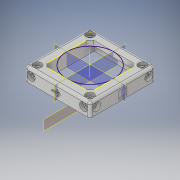
# Autodesk Inventor part: 10_Lid_v0_B
Saved by Autodesk Inventor 2019 (Build 230136000, 136)
## iProperties
Created: 2018-05-19
Part Number: 10_Lid_v0_B
Material: Generisch
Document SubType Name: Modeling
Designer: diederichbenedict
Density: 1 g/cm^3
Appearance: Vorgabe
Author: diederichbenedict
Autodesk Inventor part; units mm, degrees
ref_plane "YZ Plane" through (0, 0, 0) normal (1, 0, 0) x (0, 1, 0)
ref_plane "XZ Plane" through (0, 0, 0) normal (0, 1, 0) x (-1, 0, 0)
sketch "Skizze1" plane through (0, 0, 0) normal (0, 0, 1) x (1, 0, 0)
  line L0 (-3.2746, 3.2746) -> (46.5254, 3.2746)
  line L1 (46.5254, 3.2746) -> (46.5254, -46.5254)
  line L2 (46.5254, -46.5254) -> (-3.2746, -46.5254)
  line L3 (-3.2746, -46.5254) -> (-3.2746, 3.2746)
  line L4 (-3.2746, 3.2746) -> (46.5254, -46.5254) construction
  line L5 (46.5254, 3.2746) -> (-3.2746, -46.5254) construction
  line L6 (6.7254, -3.7254) -> (36.5254, -3.7254)
  line L7 (39.5254, -6.7254) -> (39.5254, -36.5254)
  line L8 (36.5254, -39.5254) -> (6.7254, -39.5254)
  line L9 (3.7254, -36.5254) -> (3.7254, -6.7254)
  line L10 (3.7254, -3.7254) -> (39.5254, -39.5254) construction
  line L11 (39.5254, -3.7254) -> (3.7254, -39.5254) construction
  line L12 (36.5254, -39.5254) -> (39.5254, -36.5254)
  line L13 (6.7254, -39.5254) -> (3.7254, -36.5254)
  line L14 (3.7254, -6.7254) -> (6.7254, -3.7254)
  line L15 (36.5254, -3.7254) -> (39.5254, -6.7254)
  line L16 (6.9985, -0.5594) -> (36.2523, -0.5594) projected
  line L17 (36.2523, -0.5594) -> (36.2523, 3.2746) projected
  line L18 (36.2523, 3.2746) -> (6.9985, 3.2746) projected
  line L19 (6.9985, 3.2746) -> (6.9985, -0.5594) projected
  point P0 (21.6254, -21.6254)
  point P1 (21.6254, -21.6254)
  dimension "d17" = 35.8
  dimension "d18" = 35.8
  dimension "d19" = 3
  dimension "d20" = 3
  dimension "d21" = 3
  dimension "d22" = 3
  dimension "d23" = 3
  dimension "d24" = 3
  dimension "d25" = 3
  dimension "d26" = 3
  constraints: 32 end point, 8 point on line, 5 midpoint, 4 parallel, 2 horizontal, 2 perpendicular
  measures "d17" distance of L10.end L11.end
  measures "d18" distance of L11.start L10.end
  measures "d19" distance of L8.start L10.end
  measures "d20" distance of L7.end L10.end
  measures "d21" distance of L8.end L11.end
  measures "d22" distance of L9.start L11.end
  measures "d23" distance of L9.end L10.start
  measures "d24" distance of L6.start L10.start
  measures "d25" distance of L6.end L11.start
  measures "d26" distance of L7.start L11.start
extrude "Extrusion1" add sketch "Skizze1" along normal blind 10.3
sketch "Skizze2" plane through (0, 0, 10.3) normal (0, 0, 1) x (1, 0, 0)
  arc A0 (41.4389, -3.1137) -> (40.137, -1.8118) centre (41.6254, -1.6254) ccw projected
  arc A1 (40.137, -41.4389) -> (41.4389, -40.137) centre (41.6254, -41.6254) ccw projected
  arc A2 (1.8118, -40.137) -> (3.1137, -41.4389) centre (1.6254, -41.6254) ccw projected
  arc A3 (3.1137, -1.8118) -> (1.8118, -3.1137) centre (1.6254, -1.6254) ccw projected
hole "Bohrung1" at (41.6254, -41.6254, 10.3) at (1.6254, -41.6254, 10.3) at (1.6254, -1.6254, 10.3) at (41.6254, -1.6254, 10.3) direction (0, 0, -1) diameter 3 end through all counterbore diameter 6 counterbore depth 2.5
fillet "Rundung1" radius 2 8 edges at (21.6254, -46.5254, 10.3) (-3.2746, -21.6254, 10.3) (21.6254, 3.2746, 10.3) (46.5254, -21.6254, 10.3) (46.5254, 3.2746, 5.15) (46.5254, -46.5254, 5.15) (-3.2746, -46.5254, 5.15) (-3.2746, 3.2746, 5.15)
sketch "Skizze3" plane through (-1.2746, -46.5254, 0) normal (0, -1, 0) x (1, 0, 0)
  line L0 (45.8, -37.7) -> (43.681, -37.7) construction
  line L1 (45.8, -35.7954) -> (45.8, -37.7) construction
  arc A0 (43.681, -37.7) -> (45.8, -35.7954) centre (42.9, -34.7) ccw projected
  line L2 (42.9, -36) -> (2.9, -36) construction
  line L3 (2.9, -36) -> (2.9, 5.3) construction
  line L4 (2.9, 5.3) -> (42.9, 5.3) construction
  line L5 (42.9, 5.3) -> (42.9, -36) construction
  dimension "d40" = 40
  dimension "d42" = 40
  constraints: 8 end point, 2 parallel, 1 horizontal, 1 perpendicular
  measures "d40" distance of L3.end L4.end
  measures "d42" distance from line of L4 A0.centre
sketch "Skizze4" plane through (0, 0, 10.3) normal (0, 0, 1) x (1, 0, 0)
  line L0 (36.5254, -39.5254) -> (6.7254, -39.5254) projected
  line L1 (39.5254, -6.7254) -> (39.5254, -36.5254) projected
  line L2 (3.7254, -36.5254) -> (3.7254, -6.7254) projected
  circle A0 centre (21.6254, -21.6254) radius 17.9
  point P0 (0, 0)
  constraints: 3 tangent, 1 centre point
ref_plane "Arbeitsebene1" through (3.7254, -5.5842, -33.1) normal (1, 0, 0) x (0, 1, 0)
sketch "Skizze5" plane through (3.7254, -5.5842, -33.1) normal (1, 0, 0) x (0, 1, 0)
  line L0 (-36.1071, 36.3288) -> (-36.1071, 0.4712) construction
  line L1 (-36.1071, 0.4712) -> (-33.9699, -1.666) construction
  line L2 (-33.9699, -1.666) -> (1.8877, -1.666) construction
  line L3 (1.8877, -1.666) -> (4.0249, 0.4712) construction
  line L4 (4.0249, 0.4712) -> (4.0249, 36.3288) construction
  line L5 (4.0249, 36.3288) -> (1.8877, 38.466) construction
  line L6 (1.8877, 38.466) -> (-33.9699, 38.466) construction
  line L7 (-33.9699, 38.466) -> (-36.1071, 36.3288) construction
  circle A0 centre (-1.0412, 3.4) radius 3.2639 construction
  circle A1 centre (-31.0411, 3.4) radius 3.2639 construction
  circle A2 centre (-1.0412, 33.4) radius 3.2639 construction
  circle A3 centre (-31.0411, 33.4) radius 3.2639 construction
  circle A4 centre (-16.0411, 18.4) radius 13.3985 construction
  line L8 (-34.3841, -2.666) -> (-37.1071, 0.057)
  line L9 (-37.1071, 0.057) -> (-37.1071, 36.743)
  line L10 (-37.1071, 36.743) -> (-34.3841, 39.466)
  line L11 (-34.3841, 39.466) -> (2.3019, 39.466)
  line L12 (2.3019, 39.466) -> (5.0249, 36.743)
  line L13 (5.0249, 36.743) -> (5.0249, 0.057)
  line L14 (5.0249, 0.057) -> (2.3019, -2.666)
  line L15 (2.3019, -2.666) -> (-34.3841, -2.666)
  point P0 (5.5842, 33.1)
  dimension "d27" = 1
  constraints: 16 end point, 7 other
  measures "d27" distance between parallel lines of L1 L8
ref_plane "Arbeitsebene2" through (39.5254, -37.6665, -43) normal (-1, 0, 0) x (0, 0, 1)
extrude "Extrusion3" cut sketch "Skizze5" along normal up to surface (35.8 mm away)
hole "Bohrung2" at (41.6254, -46.5254, 5.3) at (1.6254, -46.5254, 5.3) direction (0, 1, 0) diameter 3.2 depth 15 tip angle 118 counterbore diameter 6.2 counterbore depth 2.5
pattern_circular "Runde Anordnung2" count 4 over 360 about axis through (21.6254, -21.6254, 10.3) along (0, 0, 1) of "Bohrung2"
sketch "Sketch6" plane through (46.5254, -44.5254, 0) normal (1, 0, 0) x (0, 0, -1)
  arc A0 (-8.3, 42.119) -> (-4.2046, 45.8) centre (-5.3, 42.9) ccw projected
  line L0 (-8.3, 3.681) -> (-8.3, 42.119) projected
  arc A1 (-4.2046, 0) -> (-8.3, 3.681) centre (-5.3, 2.9) ccw projected
  line L1 (0, 0) -> (-4.2046, 0) projected
  line L2 (0, 45.8) -> (0, 0) projected
  line L3 (-4.2046, 45.8) -> (0, 45.8) projected
  line L4 (-1.2046, 25.9) -> (-7.2046, 25.9)
  line L5 (-7.2046, 25.9) -> (-7.2046, 19.9)
  line L6 (-1.2046, 19.9) -> (-1.2046, 25.9)
  line L7 (-8.3, 22.9) -> (0, 22.9) construction
  line L8 (-4.2046, 22.9) -> (-4.2046, 45.8) construction
  line L9 (-4.2046, 22.9) -> (-4.2046, 0) construction
  line L10 (-1.2046, 19.9) -> (-7.2046, 19.9)
  point P0 (0, 44.5254)
  dimension "d49" = 6
  dimension "d50" = 6
  constraints: 14 end point, 2 midpoint, 2 parallel, 2 perpendicular, 1 horizontal, 1 point on line, 2 other
  measures "d49" distance of L5.start L5.end
  measures "d50" distance of L6.end L5.start
extrude "Extrusion4" cut sketch "Sketch6" against normal blind 1 contours L6 L10 L5 L4
ref_plane "Work Plane3" through (21.6254, -21.6254, 10.3) normal (-1, 0, 0) x (0, 0, 1)
mirror "Mirror1" about plane through (21.6254, -21.6254, 10.3) normal (-1, 0, 0) of "Extrusion4"
sketch "Sketch8" plane through (-1.2746, -46.5254, 0) normal (0, -1, 0) x (1, 0, 0)
  line L0 (22.234, 6.3594) -> (23.7514, 4.842)
  line L1 (25.6112, 4.2046) -> (22.9019, 1.4953)
  line L2 (22.234, 2.1632) -> (23.638, 3.5671)
  line L3 (23.7514, 4.842) -> (18.7736, 4.842)
  line L4 (18.7736, 3.5671) -> (23.638, 3.5671)
  line L5 (18.7736, 4.842) -> (18.7736, 3.5671)
  line L6 (22.9019, 1.4953) -> (22.234, 2.1632)
  line L7 (25.6112, 4.2046) -> (22.8452, 6.9705)
  line L8 (22.8452, 6.9705) -> (22.234, 6.3594)
  arc A0 (42.119, 8.3) -> (45.8, 4.2046) centre (42.9, 5.3) ccw projected
  line L9 (3.681, 8.3) -> (42.119, 8.3) projected
  arc A1 (0, 4.2046) -> (3.681, 8.3) centre (2.9, 5.3) ccw projected
  line L10 (0, 0) -> (0, 4.2046) projected
  line L11 (45.8, 0) -> (0, 0) projected
  line L12 (45.8, 4.2046) -> (45.8, 0) projected
  line L13 (22.9, 8.3) -> (22.9, 0) construction
  line L14 (5, 0) -> (40.8, 0) construction
  line L15 (45.8, 0) -> (45.8, 4.2046) construction
  line L16 (0, 4.2046) -> (45.8, 4.2046) construction
  point P0 (1.2746, 0)
  point P1 (21.3799, 4.0952)
  constraints: 22 end point, 5 perpendicular, 2 midpoint, 1 horizontal, 1 parallel, 1 point on line
ref_plane "Work Plane4" through (21.6254, -21.6254, 10.3) normal (0, 1, 0) x (0, 0, 1)
extrude "Extrusion5" cut sketch "Sketch8" against normal blind 1 contours L8 L7 L1 L6 L2 L4 L5 L3 L0
mirror "Mirror2" about plane through (21.6254, -21.6254, 10.3) normal (0, 1, 0) of "Extrusion5"
equation "\"d20\" = d19"
equation "\"d21\" = d19"
equation "\"d22\" = d21"
equation "\"d23\" = d19"
equation "\"d24\" = d23"
equation "\"d25\" = d19"
equation "\"d26\" = d25"
equation "\"d50\" = d49"
